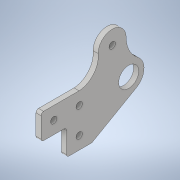
# Autodesk Inventor part: KettenBlech_Oben_Hinten
Saved by Autodesk Inventor 2021.3 (Build 253353000, 353)
## iProperties
Created: 2020-01-07
Part Number: KettenBlech_Oben_Hinten
Material: Generisch
Document SubType Name: Modeling
Designer: kaebi
Density: 1 g/cm^3
Appearance: Vorgabe
Description: Aufnahme Umlenkung (Bestand)
Stock Number: -
Author: kaebi
Autodesk Inventor part; units mm, degrees
ref_plane "YZ Plane" through (0, 0, 0) normal (1, 0, 0) x (0, 1, 0)
ref_plane "XZ Plane" through (0, 0, 0) normal (0, 1, 0) x (-1, 0, 0)
ref_plane "XY Plane" through (0, 0, 0) normal (0, 0, 1) x (1, 0, 0)
sketch "Skizze1" plane through (0, 0, 0) normal (1, 0, 0) x (0, 1, 0)
  line L0 (10, 30) -> (-10, 30)
  line L1 (-10, 30) -> (-10, 10)
  line L2 (-10, 10) -> (-30.5, 10)
  line L3 (-30.5, 10) -> (-30.5, -10)
  line L4 (-30.5, -10) -> (-30.5, -10)
  line L5 (-30.5, -10) -> (-10.5, -45)
  line L6 (10, 0) -> (10, 30)
  arc A0 (28, -37) -> (27.8513, -15.001) centre (28, -26) ccw
  arc A1 (10, 0) -> (27.8513, -15.001) centre (26, 0.918) ccw
  arc A2 (-10.5, -45) -> (9.7132, -46.2044) centre (0, -39) ccw
  arc A3 (28, -37) -> (9.7132, -46.2044) centre (28, -59.7678) ccw
  point P0 (0, 0)
  point P1 (-30.5, 0)
  point P2 (0, 30)
  dimension "d0" = 20
  dimension "d1" = 20
  dimension "d3" = 40
  dimension "d6" = 0
  dimension "d41" = 20
  dimension "d43" = 22
  dimension "d45" = 18
  dimension "d56" = 16
  dimension "d60" = 45
  dimension "d61" = 39
  dimension "d62" = 10
  dimension "d63" = 18
  dimension "d67" = 26
  dimension "d68" = 0.918
  constraints: 14 end point, 8 point on circle, 4 centre point, 3 perpendicular, 3 tangent, 2 midpoint, 1 horizontal, 1 horizontal alignment, 1 vertical, 1 vertical alignment
  measures "d0" distance of L2.end L3.end
  measures "d1" distance of L0.start L0.end
  measures "d3" distance between parallel lines of L4 L0
  measures "d6" distance of L3.end L4.end
  measures "d41" distance from line of L3 L5.end
  measures "d43" diameter of A0
  measures "d45" distance from line of A0.centre L6
  measures "d56" distance from line of L6 A1.centre
  measures "d60" vertical distance of point (0, 0) L5.end
  measures "d61" distance of A2.centre point (0, 0)
  measures "d62" distance from line of A2.centre L6
  measures "d63" distance from line of L6 A3.centre
  measures "d67" vertical distance of point (0, 0) A0.centre
  measures "d68" vertical distance of point (0, 0) A1.centre
extrude "Extrusion1" add sketch "Skizze1" along normal mid plane 4
fillet "Rundung1" radius 2 5 edges at (0, 10, 30) (0, -10, 30) (0, -10, 10) (0, -30.5, 10) (0, -30.5, -10)
sketch "Skizze2" plane through (2, 0, 0) normal (1, 0, 0) x (0, 0, -1)
  circle A0 centre (-20, 0) radius 2.5
  circle A1 centre (0, 0) radius 2.5
  circle A2 centre (0, -20.5) radius 2.5
  circle A3 centre (39, 0) radius 7.9
  line L0 (-8, -30.5) -> (9.4689, -30.5) projected
  line L1 (-30, 8) -> (-30, -8) projected
  line L2 (0, 10) -> (-28, 10) projected
  circle A4 centre (26, 28) radius 2.5
  arc A5 (37, 28) -> (15.001, 27.8513) centre (26, 28) ccw projected
  point P0 (0, 0)
  point P1 (0.7344, -30.5)
  dimension "d10" = 5
  dimension "d11" = 5
  dimension "d12" = 5
  dimension "d13" = 10
  dimension "d14" = 20
  dimension "d15" = 10
  dimension "d16" = 15.8
  dimension "d58" = 0
  dimension "d64" = 5
  dimension "d69" = 39
  constraints: 5 centre point, 1 coincident, 1 concentric, 1 horizontal alignment, 1 midpoint
  measures "d10" diameter of A0
  measures "d11" diameter of A1
  measures "d12" diameter of A2
  measures "d13" distance from line of L1 A0.centre
  measures "d14" distance of A0.centre A1.centre
  measures "d15" distance from line of L0 A2.centre
  measures "d16" diameter of A3
  measures "d58" vertical distance of A3.centre point (0, 0)
  measures "d64" diameter of A4
  measures "d69" distance of A3.centre point (0, 0)
extrude "Extrusion2" cut sketch "Skizze2" against normal through all
